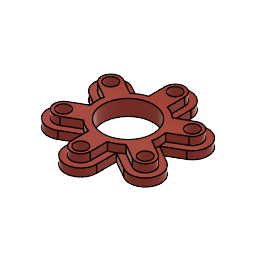
29aug (Autodesk Fusion 360 design; units mm, degrees)
part number: 2026-08-29-10-52-39-969
Autodesk Fusion 360 part; units mm, degrees
note: some values were not read from the file. Set by a fixed rule: the direction of a hole.
sketch "Sketch1" plane through (0, 0, 0) normal (0, 1, 0) x (1, 0, 0)
  circle A0 centre (0, 0) radius 16
  circle A1 centre (0, 0) radius 30 construction
  arc A2 (-6, -30) -> (6, -30) centre (0, -30) ccw
  arc A3 (6, 30) -> (-6, 30) centre (0, 30) ccw
  arc A4 (-10, -30) -> (10, -30) centre (0, -30) ccw
  arc A5 (10, 30) -> (-10, 30) centre (0, 30) ccw
  circle A6 centre (0, 0) radius 20
  line L0 (-10, 30) -> (-10, 17.3205)
  line L1 (-10, -17.3205) -> (-10, -30)
  line L2 (-6, 30) -> (-6, 19.0788)
  line L3 (-6, -19.0788) -> (-6, -30)
  line L4 (0, 30) -> (0, 20) construction
  line L5 (0, -16) -> (0, -30) construction
  line L6 (6, -30) -> (6, -19.0788)
  line L7 (6, 19.0788) -> (6, 30)
  line L8 (10, -30) -> (10, -17.3205)
  line L9 (10, 17.3205) -> (10, 30)
  line L10 (-20, 0) -> (-30.9808, -6.3397)
  line L11 (-19.5227, -4.3432) -> (-28.9808, -9.8038)
  line L12 (-22.9808, -20.1962) -> (-13.5227, -14.7355)
  line L13 (-20.9808, -23.6603) -> (-10, -17.3205)
  arc A7 (-30.9808, -6.3397) -> (-20.9808, -23.6603) centre (-25.9808, -15) ccw
  arc A8 (-28.9808, -9.8038) -> (-22.9808, -20.1962) centre (-25.9808, -15) ccw
  line L14 (20, 0) -> (30.9808, 6.3397)
  line L15 (19.5227, 4.3432) -> (28.9808, 9.8038)
  line L16 (22.9808, 20.1962) -> (13.5227, 14.7355)
  line L17 (20.9808, 23.6603) -> (10, 17.3205)
  arc A9 (30.9808, 6.3397) -> (20.9808, 23.6603) centre (25.9808, 15) ccw
  arc A10 (28.9808, 9.8038) -> (22.9808, 20.1962) centre (25.9808, 15) ccw
  line L18 (10, -17.3205) -> (20.9808, -23.6603)
  line L19 (13.5227, -14.7355) -> (22.9808, -20.1962)
  line L20 (28.9808, -9.8038) -> (19.5227, -4.3432)
  line L21 (30.9808, -6.3397) -> (20, 0)
  arc A11 (20.9808, -23.6603) -> (30.9808, -6.3397) centre (25.9808, -15) ccw
  arc A12 (22.9808, -20.1962) -> (28.9808, -9.8038) centre (25.9808, -15) ccw
  line L22 (-10, 17.3205) -> (-20.9808, 23.6603)
  line L23 (-13.5227, 14.7355) -> (-22.9808, 20.1962)
  line L24 (-28.9808, 9.8038) -> (-19.5227, 4.3432)
  line L25 (-30.9808, 6.3397) -> (-20, 0)
  arc A13 (-20.9808, 23.6603) -> (-30.9808, 6.3397) centre (-25.9808, 15) ccw
  arc A14 (-22.9808, 20.1962) -> (-28.9808, 9.8038) centre (-25.9808, 15) ccw
  dimension "d1" = 32
  dimension "d2" = 60
  dimension "d3" = 12
  dimension "d5" = 40
  dimension "d7" = 360
  constraint coincident A0.centre A1.centre
  constraint tangent A2 L3
  constraint tangent A2 L6
  constraint parallel L2 L7
  constraint tangent A3 L7
  constraint tangent A3 L2
  constraint coincident A1 A2.centre
  constraint vertical L4
  constraint coincident A1 A3.centre
  constraint concentric A2 A4
  constraint concentric A3 A5
  constraint tangent A5 L9
  constraint tangent A5 L0
  constraint tangent A4 L1
  constraint tangent A4 L8
  constraint coincident A6 L0.end
  constraint collinear L0 L1
  constraint coincident A6 L2.end
  constraint collinear L2 L3
  constraint coincident A6 L4.end
  constraint collinear L4 L5
  constraint coincident A6 L7.start
  constraint collinear L6 L7
  constraint coincident A6 L9.start
  constraint collinear L8 L9
  constraint coincident A0 L5.start
  constraint coincident A6 L1.start
  constraint coincident A6 L3.start
  constraint coincident A6 L6.end
  constraint coincident A6 L8.end
  measures "d1" diameter of A0
  measures "d2" diameter of A1
  measures "d3" diameter of A2
  measures "d5" diameter of A6
extrude "Extrude1" add sketch "Sketch1" along normal blind 10 contours A2 A6 L3 L6 | A6 | A6 L11 L12 A8 | A6 L19 L20 A12 | A6 L23 L24 A14 | A6 L15 L16 A10 | A3 A6 L2 L7
extrude "Extrude2" add sketch "Sketch1" along normal blind 5 contours A2 A4 A6 L1 L3 L6 L8 | A6 L10 L11 L12 L13 A7 A8 | A6 L18 L19 L20 L21 A11 A12 | A6 L22 L23 L24 L25 A13 A14 | A6 L14 L15 L16 L17 A9 A10 | A3 A5 A6 L0 L2 L7 L9
hole "Hole1" at (0, 0, -30) direction (0, 1, 0) diameter 8 end through all
pattern_circular "C-Pattern1" count 6 over 360 about axis through (0, 1.75, 0) along (0, 1, 0) of "Hole1"
